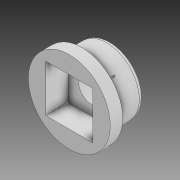
# Autodesk Inventor part: HD_BearingShaft1
Saved by Autodesk Inventor 2020 (Build 240168000, 168)
## iProperties
Created: 2021-03-21
Part Number: HD_BearingShaft1
Material: Generic
Document SubType Name: Modeling
Designer: DDeGo
Density: 1 g/cm^3
Appearance: Default
Author: DDeGo
Autodesk Inventor part; units mm, degrees
ref_plane "YZ Plane" through (0, 0, 0) normal (1, 0, 0) x (0, 1, 0)
ref_plane "XZ Plane" through (0, 0, 0) normal (0, 1, 0) x (-1, 0, 0)
ref_plane "XY Plane" through (0, 0, 0) normal (0, 0, 1) x (1, 0, 0)
sketch "Sketch1" plane through (0, 0, 0) normal (1, 0, 0) x (0, 1, 0)
  line L0 (0, 0) -> (1.6, 0) construction
  line L1 (1.6, 0) -> (4.95, 0)
  line L2 (4.95, 0) -> (4.95, -1.5)
  line L3 (4.95, -1.5) -> (3.95, -1.5)
  line L4 (3.95, -1.5) -> (3.95, -5)
  line L5 (3.95, -5) -> (1.6, -5)
  line L6 (1.6, -5) -> (1.6, 0)
  line L7 (0, 0) -> (0, -13.7466) construction
  dimension "d0" = 1.6
  dimension "d1" = 3.95
  dimension "d2" = 1
  dimension "d3" = 1.5
  dimension "d4" = 3.5
  constraints: 16 end point, 4 perpendicular, 2 vertical, 1 horizontal, 1 point on line
  measures "d0" distance between parallel lines of L7 L6
  measures "d1" distance between parallel lines of L7 L4
  measures "d2" distance between parallel lines of L4 L2
  measures "d3" distance between parallel lines of L1 L3
  measures "d4" distance of L3.end L4.end
revolve "Revolution1" add sketch "Sketch1" angle 360 about axis through (0, 0, 0) along (0, 0, -1)
sketch "Sketch2" plane through (0, 0, 0) normal (0, 0, 1) x (1, 0, 0)
  line L0 (2.85, -2.85) -> (-2.85, -2.85)
  line L1 (-2.85, -2.85) -> (-2.85, 2.85)
  line L2 (-2.85, 2.85) -> (2.85, 2.85)
  line L3 (2.85, 2.85) -> (2.85, -2.85)
  line L4 (2.85, -2.85) -> (-2.85, 2.85) construction
  line L5 (-2.85, -2.85) -> (2.85, 2.85) construction
  point P0 (0, 0)
  dimension "d6" = 5.7
  constraints: 12 end point, 2 midpoint, 2 parallel, 2 perpendicular, 1 horizontal
  measures "d6" distance of L0.end L1.end
extrude "Extrusion1" cut sketch "Sketch2" against normal blind 2.7
fillet "Fillet1" radius 0.5 2 edges at (0, -3.95, -5) (0, -1.6, -5)
body "Solid1"
